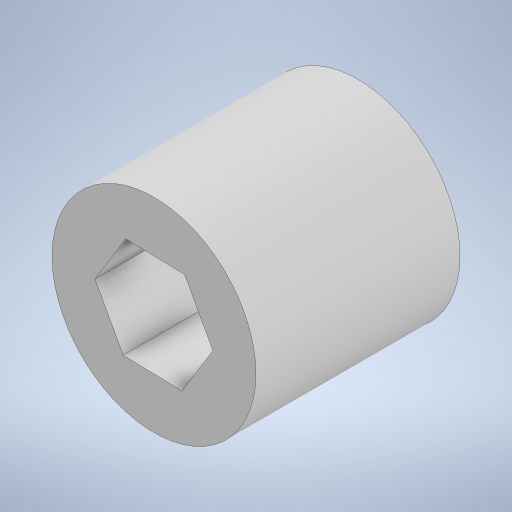
# Autodesk Inventor part: 4-bar intake (1'') spacer
Saved by Autodesk Inventor 2023 (Build 270158030, 158C)
## iProperties
Created: 2022-07-19
Part Number: 4-bar intake (1'') spacer
Material: Generic
Document SubType Name: Modeling
Designer: rm0990889
Density: 1 g/cm^3
Appearance: Default
Author: rm0990889
Autodesk Inventor part; units mm, degrees
ref_plane "YZ Plane" through (0, 0, 0) normal (1, 0, 0) x (0, 1, 0)
ref_plane "XZ Plane" through (0, 0, 0) normal (0, 1, 0) x (-1, 0, 0)
ref_plane "XY Plane" through (0, 0, 0) normal (0, 0, 1) x (1, 0, 0)
sketch "Sketch1" plane through (0, 0, 0) normal (0, 0, 1) x (1, 0, 0)
  circle A0 centre (0, 0) radius 6.35
  line L0 (7.3298, -0.1918) -> (3.4988, -6.4437)
  line L1 (3.4988, -6.4437) -> (-3.831, -6.2519)
  line L2 (-3.831, -6.2519) -> (-7.3298, 0.1918)
  line L3 (-7.3298, 0.1918) -> (-3.4988, 6.4437)
  line L4 (-3.4988, 6.4437) -> (3.831, 6.2519)
  line L5 (3.831, 6.2519) -> (7.3298, -0.1918)
  circle A1 centre (0, 0) radius 12.7
  point P0 (5.5804, 3.0301)
  dimension "d0" = 12.7
  dimension "d1" = 25.4
  constraints: 12 end point, 3 coincident, 1 centre point, 1 midpoint, 16 other
  measures "d1" diameter of A1
extrude "Extrusion1" add sketch "Sketch1" along normal blind 25.4
body "Solid1"
